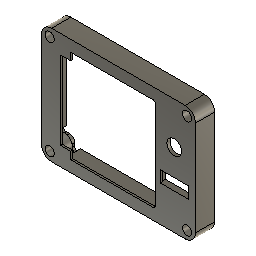
deksel groot projectdoosje v9 (Autodesk Fusion 360 design; units mm, degrees)
Autodesk Fusion 360 part; units mm, degrees
sketch "Sketch1" plane through (0, 0, 0) normal (0, 1, 0) x (1, 0, 0)
  line L0 (8, 0) -> (112, 0)
  line L1 (120, -8) -> (120, -82)
  line L2 (112, -90) -> (8, -90)
  line L3 (0, -82) -> (0, -8)
  arc A0 (0, -82) -> (8, -90) centre (8, -82) ccw
  arc A1 (8, 0) -> (0, -8) centre (8, -8) ccw
  arc A2 (120, -8) -> (112, 0) centre (112, -8) ccw
  arc A3 (112, -90) -> (120, -82) centre (112, -82) ccw
  point P0 (120, 0)
  point P1 (0, -90)
  dimension "d1" = 120
  dimension "d2" = 90
  dimension "d3" = 8
  constraint horizontal L0
  constraint vertical L1
  constraint horizontal L2
  constraint vertical L3
  constraint coincident P1 L2
  constraint coincident P1 L3
  constraint tangent L2 A0
  constraint tangent L3 A0
  constraint coincident origin L0
  constraint coincident origin L3
  constraint tangent L0 A1
  constraint tangent L3 A1
  constraint equal A0 A1
  constraint coincident P0 L0
  constraint coincident P0 L1
  constraint tangent L0 A2
  constraint tangent L1 A2
  constraint equal A0 A2
  constraint tangent L1 A3
  constraint tangent L2 A3
  constraint equal A0 A3
  measures "d1" distance of origin P0
  measures "d2" distance of origin P1
  measures "d3" radius of A0
extrude "Extrude1" add sketch "Sketch1" along normal blind 15
sketch "Sketch2" plane through (0, 0, 0) normal (0, -1, 0) x (1, 0, 0)
  arc A0 (8, 90) -> (0, 82) centre (8, 82) ccw
  line L0 (0, 82) -> (0, 8)
  arc A1 (0, 8) -> (8, 0) centre (8, 8) ccw
  line L1 (8, 0) -> (112, 0)
  arc A2 (112, 0) -> (120, 8) centre (112, 8) ccw
  line L2 (120, 8) -> (120, 82)
  arc A3 (120, 82) -> (112, 90) centre (112, 82) ccw
  line L3 (112, 90) -> (8, 90)
  line L4 (60, 0) -> (60, 90) construction
  line L5 (120, 45) -> (0, 45) construction
  point P0 (6.5, 6.5)
  point P1 (6.5, 83.5)
  point P2 (113.5, 6.5)
  point P3 (113.5, 83.5)
  dimension "d86" = 107
  dimension "d87" = 77
  constraint midpoint L1 L4.start
  constraint midpoint L3 L4.end
  constraint midpoint L2 L5.start
  constraint midpoint L0 L5.end
  constraint symmetric P0 P2 L4
  constraint symmetric P2 P3 L5
  constraint symmetric P0 P1 L5
  measures "d86" distance of P0 P2
  measures "d87" distance of P2 P3
hole "Hole1" at (6.5, 0, 83.5) at (6.5, 0, 6.5) at (113.5, 0, 6.5) at (113.5, 0, 83.5) direction (0, 1, 0) diameter 4 end through all counterbore diameter 7.2 counterbore depth 5
sketch "Sketch3" plane through (0, 0, 0) normal (0, -1, 0) x (1, 0, 0)
  circle A0 centre (113.5, 6.5) radius 3.6
  circle A1 centre (6.5, 83.5) radius 3.6
  circle A2 centre (6.5, 6.5) radius 3.6
  circle A3 centre (113.5, 83.5) radius 3.6
  arc A4 (8, 90) -> (0, 82) centre (8, 82) ccw
  line L0 (0, 82) -> (0, 8)
  arc A5 (0, 8) -> (8, 0) centre (8, 8) ccw
  line L1 (8, 0) -> (112, 0)
  arc A6 (112, 0) -> (120, 8) centre (112, 8) ccw
  line L2 (120, 8) -> (120, 82)
  arc A7 (120, 82) -> (112, 90) centre (112, 82) ccw
  line L3 (112, 90) -> (8, 90)
  circle A8 centre (6.5, 6.5) radius 3
  circle A9 centre (6.5, 83.5) radius 3
  circle A10 centre (113.5, 83.5) radius 3
  circle A11 centre (113.5, 6.5) radius 3
  dimension "d18" = 6
  dimension "d19" = 6
  dimension "d20" = 6
  dimension "d21" = 6
  constraint concentric A2 A8
  constraint concentric A1 A9
  constraint concentric A3 A10
  constraint concentric A0 A11
  measures "d18" diameter of A8
  measures "d19" diameter of A9
  measures "d20" diameter of A10
  measures "d21" diameter of A11
extrude "Extrude2" cut sketch "Sketch3" against normal blind 11 contours A8 | A9 | A10 | A11
sketch "Sketch4" plane through (0, 0, 0) normal (0, -1, 0) x (1, 0, 0)
  circle A0 centre (113.5, 6.5) radius 3.6
  circle A1 centre (6.5, 83.5) radius 3.6
  circle A2 centre (6.5, 6.5) radius 3.6
  circle A3 centre (113.5, 83.5) radius 3.6
  arc A4 (8, 90) -> (0, 82) centre (8, 82) ccw
  line L0 (0, 82) -> (0, 8)
  arc A5 (0, 8) -> (8, 0) centre (8, 8) ccw
  line L1 (8, 0) -> (112, 0)
  arc A6 (112, 0) -> (120, 8) centre (112, 8) ccw
  line L2 (120, 8) -> (120, 82)
  arc A7 (120, 82) -> (112, 90) centre (112, 82) ccw
  line L3 (112, 90) -> (8, 90)
  circle A8 centre (6.5, 6.5) radius 3.5
  line L4 (4.7617, 3.3475) -> (9.6525, 8.2383)
  line L5 (3.3475, 4.7617) -> (8.2383, 9.6525)
  line L6 (60, 90) -> (60, 0) construction
  line L7 (0, 45) -> (120, 45) construction
  circle A9 centre (6.5, 83.5) radius 3.5
  line L8 (4.7617, 86.6525) -> (9.6525, 81.7617)
  line L9 (3.3475, 85.2383) -> (8.2383, 80.3475)
  line L10 (115.2383, 86.6525) -> (110.3475, 81.7617)
  line L11 (116.6525, 85.2383) -> (111.7617, 80.3475)
  circle A10 centre (113.5, 83.5) radius 3.5
  circle A11 centre (113.5, 6.5) radius 3.5
  line L12 (116.6525, 4.7617) -> (111.7617, 9.6525)
  line L13 (115.2383, 3.3475) -> (110.3475, 8.2383)
  dimension "d24" = 45
  dimension "d25" = 2
  dimension "d26" = 1
  dimension "d27" = 6.5
  dimension "d28" = 7
  constraint concentric A2 A8
  constraint coincident A2 L4.start
  constraint coincident A2 L4.end
  constraint coincident A2 L5.start
  constraint coincident A2 L5.end
  constraint parallel L4 L5
  constraint midpoint L3 L6.start
  constraint midpoint L1 L6.end
  constraint midpoint L0 L7.start
  constraint midpoint L2 L7.end
  constraint symmetric A8 L7 A9
  constraint symmetric L4.start L7 L8.start
  constraint symmetric L4.end L7 L8.end
  constraint symmetric L5.start L7 L9.start
  constraint symmetric L5.end L7 L9.end
  constraint symmetric A8 L6 A11
  constraint symmetric L4.start L6 L13.start
  constraint symmetric L4.end L6 L13.end
  constraint symmetric L5.start L6 L12.start
  constraint symmetric L5.end L6 L12.end
  constraint symmetric L6 A9 A10
  constraint symmetric L6 L8.start L10.start
  constraint symmetric L6 L8.end L10.end
  constraint symmetric L6 L9.start L11.start
  constraint symmetric L6 L9.end L11.end
  measures "d24" angle of L1 L4
  measures "d25" distance of L4 L5
  measures "d26" distance of A2.centre L4
  measures "d27" distance of L1 A2.centre
  measures "d28" diameter of A8
extrude "Extrude3" cut sketch "Sketch4" against normal through all contours A11 L12 L13 | A9 L8 L9 | A8 L4 L5 | L10 L11 A10
sketch "Sketch11" plane through (0, 15, 0) normal (0, 1, 0) x (-1, 0, 0)
  line L0 (-116.5788, 4.8354) -> (-115.4319, 5.9824)
  arc A0 (-112.9824, 8.4319) -> (-115.4319, 5.9824) centre (-113.5, 6.5) ccw
  line L1 (-112.9824, 8.4319) -> (-111.8354, 9.5788)
  arc A1 (-110.4212, 8.1646) -> (-111.8354, 9.5788) centre (-113.5, 6.5) ccw
  line L2 (-110.4212, 8.1646) -> (-111.5681, 7.0176)
  arc A2 (-114.0176, 4.5681) -> (-111.5681, 7.0176) centre (-113.5, 6.5) ccw
  line L3 (-114.0176, 4.5681) -> (-115.1646, 3.4212)
  line L4 (-111.8354, 80.4212) -> (-112.9824, 81.5681)
  arc A3 (-115.4319, 84.0176) -> (-112.9824, 81.5681) centre (-113.5, 83.5) ccw
  line L5 (-115.4319, 84.0176) -> (-116.5788, 85.1646)
  arc A4 (-115.1646, 86.5788) -> (-116.5788, 85.1646) centre (-113.5, 83.5) ccw
  line L6 (-115.1646, 86.5788) -> (-114.0176, 85.4319)
  arc A5 (-111.5681, 82.9824) -> (-114.0176, 85.4319) centre (-113.5, 83.5) ccw
  line L7 (-111.5681, 82.9824) -> (-110.4212, 81.8354)
  arc A6 (-111.8354, 80.4212) -> (-110.4212, 81.8354) centre (-113.5, 83.5) ccw
  line L8 (-8.1646, 9.5788) -> (-7.0176, 8.4319)
  arc A7 (-4.5681, 5.9824) -> (-7.0176, 8.4319) centre (-6.5, 6.5) ccw
  line L9 (-4.5681, 5.9824) -> (-3.4212, 4.8354)
  arc A8 (-4.8354, 3.4212) -> (-3.4212, 4.8354) centre (-6.5, 6.5) ccw
  line L10 (-4.8354, 3.4212) -> (-5.9824, 4.5681)
  arc A9 (-8.4319, 7.0176) -> (-5.9824, 4.5681) centre (-6.5, 6.5) ccw
  line L11 (-8.4319, 7.0176) -> (-9.5788, 8.1646)
  arc A10 (-8.1646, 9.5788) -> (-9.5788, 8.1646) centre (-6.5, 6.5) ccw
  line L12 (-3.4212, 85.1646) -> (-4.5681, 84.0176)
  arc A11 (-7.0176, 81.5681) -> (-4.5681, 84.0176) centre (-6.5, 83.5) ccw
  line L13 (-7.0176, 81.5681) -> (-8.1646, 80.4212)
  arc A12 (-9.5788, 81.8354) -> (-8.1646, 80.4212) centre (-6.5, 83.5) ccw
  line L14 (-9.5788, 81.8354) -> (-8.4319, 82.9824)
  arc A13 (-5.9824, 85.4319) -> (-8.4319, 82.9824) centre (-6.5, 83.5) ccw
  line L15 (-5.9824, 85.4319) -> (-4.8354, 86.5788)
  arc A14 (0, 82) -> (-8, 90) centre (-8, 82) ccw
  line L16 (-8, 90) -> (-112, 90)
  arc A15 (-112, 90) -> (-120, 82) centre (-112, 82) ccw
  line L17 (-120, 82) -> (-120, 8)
  arc A16 (-120, 8) -> (-112, 0) centre (-112, 8) ccw
  line L18 (-112, 0) -> (-8, 0)
  arc A17 (-8, 0) -> (0, 8) centre (-8, 8) ccw
  line L19 (0, 8) -> (0, 82)
  line L20 (-120, 45) -> (0, 45) construction
  line L21 (-60, 90) -> (-60, 0) construction
  line L22 (-118.5, 45) -> (-118.5, 79)
  line L23 (-118.5, 79) -> (-113, 79)
  line L24 (-109, 83) -> (-109, 88.5)
  line L25 (-109, 88.5) -> (-60, 88.5)
  arc A18 (-113, 79) -> (-109, 83) centre (-113, 83) ccw
  arc A19 (-116.5788, 4.8354) -> (-115.1646, 3.4212) centre (-113.5, 6.5) ccw
  arc A20 (-3.4212, 85.1646) -> (-4.8354, 86.5788) centre (-6.5, 83.5) ccw
  line L26 (-11, 88.5) -> (-60, 88.5)
  line L27 (-11, 83) -> (-11, 88.5)
  arc A21 (-11, 83) -> (-7, 79) centre (-7, 83) ccw
  line L28 (-1.5, 79) -> (-7, 79)
  line L29 (-1.5, 45) -> (-1.5, 79)
  line L30 (-118.5, 45) -> (-118.5, 11)
  line L31 (-118.5, 11) -> (-113, 11)
  arc A22 (-109, 7) -> (-113, 11) centre (-113, 7) ccw
  line L32 (-109, 7) -> (-109, 1.5)
  line L33 (-109, 1.5) -> (-60, 1.5)
  line L34 (-11, 1.5) -> (-60, 1.5)
  line L35 (-11, 7) -> (-11, 1.5)
  arc A23 (-7, 11) -> (-11, 7) centre (-7, 7) ccw
  line L36 (-1.5, 11) -> (-7, 11)
  line L37 (-1.5, 45) -> (-1.5, 11)
  dimension "d88" = 11
  dimension "d89" = 11
  dimension "d90" = 1.5
  dimension "d91" = 1.5
  dimension "d92" = 4
  constraint midpoint L17 L20.start
  constraint midpoint L19 L20.end
  constraint midpoint L16 L21.start
  constraint midpoint L18 L21.end
  constraint coincident L20 L22.start
  constraint perpendicular L20 L22
  constraint perpendicular L22 L23
  constraint perpendicular L23 L24
  constraint coincident L21 L25.end
  constraint perpendicular L21 L25
  constraint tangent L23 A18
  constraint tangent L24 A18
  constraint symmetric L21 L22.start L29.start
  constraint symmetric L21 L22.end L28.start
  constraint symmetric L21 L24.end L26.start
  constraint symmetric L21 L25.end L26.end
  constraint symmetric L21 L23.end A21.end
  constraint symmetric L21 L24.start L27.start
  constraint symmetric L21 A18 A21
  constraint symmetric L20 L22.start L30.start
  constraint symmetric L20 L22.end L30.end
  constraint symmetric L20 L24.end L32.end
  constraint symmetric L20 L25.end L33.end
  constraint symmetric L20 L23.end L31.end
  constraint symmetric L20 L24.start A22.start
  constraint symmetric L20 A18 A22
  constraint symmetric L20 L26.start L34.start
  constraint symmetric L20 L27.start L35.start
  constraint symmetric L20 A21.end A23.start
  constraint symmetric L20 A21 A23
  constraint symmetric L20 L28.start L36.start
  constraint symmetric L20 L29.start L37.start
  measures "d88" distance of L17 L24
  measures "d89" distance of L16 L23
  measures "d90" distance of L16 L25
  measures "d91" distance of L17 L22
  measures "d92" radius of A18
extrude "Extrude9" cut sketch "Sketch11" against normal up to surface (13.5 mm away) contours L22 L23 L24 L25 A18 L26 L27 A21 L28 L29 L30 L31 A22 L32 L33 L34 L35 A23 L36 L37
sketch "Sketch15" plane through (0, 1.5, 0) normal (0, 1, 0) x (-1, 0, 0)
  arc A0 (-11, 83) -> (-7, 79) centre (-7, 83) ccw
  line L0 (-11, 83) -> (-11, 88.5)
  line L1 (-11, 88.5) -> (-109, 88.5)
  line L2 (-109, 88.5) -> (-109, 83)
  arc A1 (-113, 79) -> (-109, 83) centre (-113, 83) ccw
  line L3 (-113, 79) -> (-118.5, 79)
  line L4 (-118.5, 79) -> (-118.5, 11)
  line L5 (-118.5, 11) -> (-113, 11)
  arc A2 (-109, 7) -> (-113, 11) centre (-113, 7) ccw
  line L6 (-109, 7) -> (-109, 1.5)
  line L7 (-109, 1.5) -> (-11, 1.5)
  line L8 (-11, 1.5) -> (-11, 7)
  arc A3 (-7, 11) -> (-11, 7) centre (-7, 7) ccw
  line L9 (-7, 11) -> (-1.5, 11)
  line L10 (-1.5, 11) -> (-1.5, 79)
  line L11 (-1.5, 79) -> (-7, 79)
  line L12 (-11, 1.5) -> (-109, 1.5)
  line L13 (-109, 1.5) -> (-109, 3.5)
  line L14 (-105, 3.5) -> (-14.9861, 3.5)
  line L15 (-11, 3.5) -> (-11, 1.5)
  line L16 (-118.5, 11) -> (-116.5, 11)
  line L17 (-116.5, 15) -> (-116.5, 75)
  line L18 (-116.5, 79) -> (-118.5, 79)
  line L19 (-118.5, 79) -> (-118.5, 11)
  line L20 (-11, 88.5) -> (-109, 88.5)
  line L21 (-109, 88.5) -> (-109, 86.5)
  line L22 (-105, 86.5) -> (-15, 86.5)
  line L23 (-11, 86.5) -> (-11, 88.5)
  line L24 (-1.5, 11) -> (-3.5, 11)
  line L25 (-3.5, 15) -> (-3.5, 75)
  line L26 (-3.5, 79) -> (-1.5, 79)
  line L27 (-1.5, 79) -> (-1.5, 11)
  line L28 (-5.5, 13) -> (-6, 13)
  line L29 (-13, 6) -> (-13, 3.5)
  arc A4 (-6, 13) -> (-12.9892, 5.6111) centre (-6, 6) ccw
  line L30 (-60, 3.5) -> (-60, 86.5) construction
  line L31 (-107, 6) -> (-107, 5.5)
  arc A5 (-107, 6) -> (-114, 13) centre (-114, 6) ccw
  line L32 (-114.5, 13) -> (-114, 13)
  line L33 (-3.5, 45) -> (-116.5, 45)
  line L34 (-13, 84) -> (-13, 84.5)
  arc A6 (-13, 84) -> (-6, 77) centre (-6, 84) ccw
  line L35 (-5.5, 77) -> (-6, 77)
  line L36 (-107, 84) -> (-107, 84.5)
  arc A7 (-114, 77) -> (-107, 84) centre (-114, 84) ccw
  line L37 (-114.5, 77) -> (-114, 77)
  arc A8 (-14.9861, 3.5) -> (-12.9892, 5.6111) centre (-14.9861, 5.5) ccw
  arc A9 (-5.5, 13) -> (-3.5, 15) centre (-5.5, 15) ccw
  arc A10 (-3.5, 75) -> (-5.5, 77) centre (-5.5, 75) ccw
  arc A11 (-13, 84.5) -> (-15, 86.5) centre (-15, 84.5) ccw
  arc A12 (-105, 86.5) -> (-107, 84.5) centre (-105, 84.5) ccw
  arc A13 (-114.5, 77) -> (-116.5, 75) centre (-114.5, 75) ccw
  arc A14 (-116.5, 15) -> (-114.5, 13) centre (-114.5, 15) ccw
  arc A15 (-107, 5.5) -> (-105, 3.5) centre (-105, 5.5) ccw
  dimension "d109" = 2
  dimension "d110" = 2
  dimension "d111" = 2
  dimension "d112" = 2
  dimension "d115" = 2
  dimension "d116" = 2
  dimension "d117" = 7
  dimension "d118" = 2
  constraint horizontal L12
  constraint vertical L13
  constraint horizontal L14
  constraint vertical L15
  constraint coincident L6 L13.end
  constraint coincident L7.end L8.start
  constraint horizontal L16
  constraint vertical L17
  constraint horizontal L18
  constraint vertical L19
  constraint coincident L3 L18.start
  constraint coincident L4.end L5.start
  constraint horizontal L20
  constraint vertical L21
  constraint horizontal L22
  constraint vertical L23
  constraint coincident L2 L21.end
  constraint coincident L0.end L1.start
  constraint horizontal L24
  constraint vertical L25
  constraint horizontal L26
  constraint vertical L27
  constraint coincident L11 L26.start
  constraint coincident L9.end L10.start
  constraint perpendicular L25 L28
  constraint coincident L14 L29.end
  constraint perpendicular L14 L29
  constraint tangent L28 A4
  constraint tangent L29 A4
  constraint symmetric L28.end L30 A5.end
  constraint symmetric L29.start L30 L31.start
  constraint symmetric A4 L30 A5
  constraint symmetric L28.end L33 A6.end
  constraint symmetric L29.start L33 L34.start
  constraint symmetric A4 L33 A6
  constraint symmetric L31.start L33 L36.start
  constraint symmetric A5.end L33 A7.start
  constraint symmetric A5 L33 A7
  constraint coincident L14 L30.start
  constraint tangent L14 A8
  constraint tangent A4 A8
  constraint coincident L25 L33.start
  constraint coincident L24.end L25
  constraint tangent L28 A9
  constraint tangent L25 A9
  constraint equal A8 A9
  constraint coincident L26.start L25
  constraint tangent L35 A10
  constraint tangent L25 A10
  constraint equal A8 A10
  constraint coincident L22 L30.end
  constraint coincident L23.start L22
  constraint tangent L34 A11
  constraint tangent L22 A11
  constraint equal A8 A11
  constraint coincident L21.end L22
  constraint tangent L36 A12
  constraint tangent L22 A12
  constraint equal A8 A12
  constraint coincident L17 L33.end
  constraint coincident L18.start L17
  constraint tangent L37 A13
  constraint tangent L17 A13
  constraint equal A8 A13
  constraint coincident L16.end L17
  constraint tangent L17 A14
  constraint tangent L32 A14
  constraint equal A8 A14
  constraint coincident L13.end L14
  constraint tangent L14 A15
  constraint tangent L31 A15
  constraint equal A8 A15
  measures "d109" distance of L12 L14
  measures "d110" distance of L17 L19
  measures "d111" distance of L20 L22
  measures "d112" distance of L25 L27
  measures "d115" distance of L8 L29
  measures "d116" distance of L9 L28
  measures "d117" radius of A4
  measures "d118" radius of A8
extrude "Extrude13" add sketch "Sketch15" along normal up to surface (10 mm away)
fillet "Fillet2" radius 3 8 edges at (11, 13.25, 1.5) (1.5, 13.25, 11) (109, 13.25, 1.5) (118.5, 13.25, 11) (109, 13.25, 88.5) (118.5, 13.25, 79) (11, 13.25, 88.5) (1.5, 13.25, 79)
sketch "Sketch16" plane through (0, 1.5, 0) normal (0, 1, 0) x (-1, 0, 0)
  arc A0 (-107, 6) -> (-114, 13) centre (-114, 6) ccw
  line L0 (-107, 6) -> (-107, 5.5)
  arc A1 (-107, 5.5) -> (-105, 3.5) centre (-105, 5.5) ccw
  line L1 (-105, 3.5) -> (-14.9861, 3.5)
  arc A2 (-14.9861, 3.5) -> (-12.9892, 5.6111) centre (-14.9861, 5.5) ccw
  arc A3 (-6, 13) -> (-12.9892, 5.6111) centre (-6, 6) ccw
  line L2 (-6, 13) -> (-5.5, 13)
  arc A4 (-5.5, 13) -> (-3.5, 15) centre (-5.5, 15) ccw
  line L3 (-3.5, 15) -> (-3.5, 75)
  arc A5 (-3.5, 75) -> (-5.5, 77) centre (-5.5, 75) ccw
  line L4 (-5.5, 77) -> (-6, 77)
  arc A6 (-13, 84) -> (-6, 77) centre (-6, 84) ccw
  line L5 (-13, 84) -> (-13, 84.5)
  arc A7 (-13, 84.5) -> (-15, 86.5) centre (-15, 84.5) ccw
  line L6 (-15, 86.5) -> (-105, 86.5)
  arc A8 (-105, 86.5) -> (-107, 84.5) centre (-105, 84.5) ccw
  line L7 (-107, 84.5) -> (-107, 84)
  arc A9 (-114, 77) -> (-107, 84) centre (-114, 84) ccw
  line L8 (-114, 77) -> (-114.5, 77)
  arc A10 (-114.5, 77) -> (-116.5, 75) centre (-114.5, 75) ccw
  line L9 (-116.5, 75) -> (-116.5, 15)
  arc A11 (-116.5, 15) -> (-114.5, 13) centre (-114.5, 15) ccw
  line L10 (-114.5, 13) -> (-114, 13)
  line L11 (-104.5, 86.5) -> (-15.5, 86.5)
  line L12 (-15.5, 86.5) -> (-15.5, 85)
  line L13 (-15.5, 85) -> (-104.5, 85)
  line L14 (-104.5, 85) -> (-104.5, 86.5)
  line L15 (-3.5, 74.5) -> (-5, 74.5)
  line L16 (-5, 74.5) -> (-5, 15.5)
  line L17 (-5, 15.5) -> (-3.5, 15.5)
  line L18 (-3.5, 15.5) -> (-3.5, 74.5)
  line L19 (-15.5, 3.5) -> (-104.5, 3.5)
  line L20 (-104.5, 3.5) -> (-104.5, 5)
  line L21 (-104.5, 5) -> (-15.5, 5)
  line L22 (-15.5, 5) -> (-15.5, 3.5)
  line L23 (-116.5, 74.5) -> (-115, 74.5)
  line L24 (-115, 74.5) -> (-115, 15.5)
  line L25 (-115, 15.5) -> (-116.5, 15.5)
  line L26 (-116.5, 15.5) -> (-116.5, 74.5)
  line L27 (-103.8997, 85) -> (-104.5, 85)
  line L28 (-115, 74.5) -> (-115, 74)
  line L29 (-115, 45) -> (-5, 45) construction
  line L30 (-60, 85) -> (-60, 5) construction
  dimension "d121" = 1.5
  dimension "d122" = 12
  dimension "d123" = 12
  dimension "d124" = 1.5
  dimension "d125" = 12
  dimension "d126" = 12
  dimension "d127" = 12
  dimension "d128" = 1.5
  dimension "d129" = 12
  dimension "d130" = 1.5
  dimension "d131" = 12
  dimension "d132" = 12
  constraint horizontal L11
  constraint vertical L12
  constraint horizontal L13
  constraint vertical L14
  constraint coincident L6 L11.start
  constraint horizontal L15
  constraint vertical L16
  constraint horizontal L17
  constraint vertical L18
  constraint coincident L3 L15.start
  constraint horizontal L19
  constraint vertical L20
  constraint horizontal L21
  constraint vertical L22
  constraint coincident L1 L19.start
  constraint horizontal L23
  constraint vertical L24
  constraint horizontal L25
  constraint vertical L26
  constraint coincident L9 L23.start
  constraint horizontal L27
  constraint perpendicular L23 L28
  constraint midpoint L24 L29.start
  constraint midpoint L16 L29.end
  constraint midpoint L13 L30.start
  constraint midpoint L21 L30.end
  measures "d121" distance of L11 L13
  measures "d122" distance of L9 L14
  measures "d123" distance of L3 L12
  measures "d124" distance of L16 L18
  measures "d125" distance of L11 L15
  measures "d126" distance of L1 L17
  measures "d127" distance of L18 L22
  measures "d128" distance of L19 L21
  measures "d129" distance of L9 L19.end
  measures "d130" distance of L24 L26
  measures "d131" distance of L19 L24.end
  measures "d132" distance of L11 L23.end
extrude "Extrude14" add sketch "Sketch16" along normal up to surface (13.5 mm away) contours L1 L19 L20 L21 L22 | L9 L23 L24 L25 L26 L28 | L3 L15 L16 L17 L18 | L6 L11 L12 L13 L14 L27
sketch "Sketch17" plane through (0, 0, 0) normal (0, -1, 0) x (1, 0, 0)
  circle A0 centre (113.5, 6.5) radius 3.6
  circle A1 centre (6.5, 83.5) radius 3.6
  circle A2 centre (6.5, 6.5) radius 3.6
  circle A3 centre (113.5, 83.5) radius 3.6
  arc A4 (8, 90) -> (0, 82) centre (8, 82) ccw
  line L0 (0, 82) -> (0, 8)
  arc A5 (0, 8) -> (8, 0) centre (8, 8) ccw
  line L1 (8, 0) -> (112, 0)
  arc A6 (112, 0) -> (120, 8) centre (112, 8) ccw
  line L2 (120, 8) -> (120, 82)
  arc A7 (120, 82) -> (112, 90) centre (112, 82) ccw
  line L3 (112, 90) -> (8, 90)
  line L4 (15, 81.25) -> (87, 81.25)
  line L5 (89, 79.25) -> (89, 10.75)
  line L6 (87, 8.75) -> (15, 8.75)
  line L7 (15, 8.75) -> (15, 81.25)
  line L8 (15, 81.25) -> (23, 81.25)
  line L9 (23, 81.25) -> (23, 75.5)
  line L10 (23, 75.5) -> (15, 75.5)
  line L11 (15, 75.5) -> (15, 81.25)
  line L12 (15, 8.75) -> (23, 8.75)
  line L13 (23, 8.75) -> (23, 14.5)
  line L14 (23, 14.5) -> (15, 14.5)
  line L15 (15, 14.5) -> (15, 8.75)
  arc A8 (87, 8.75) -> (89, 10.75) centre (87, 10.75) ccw
  arc A9 (89, 79.25) -> (87, 81.25) centre (87, 79.25) ccw
  line L16 (0, 45) -> (120, 45) construction
  point P0 (89, 8.75)
  dimension "d140" = 72.5
  dimension "d141" = 74
  dimension "d143" = 8
  dimension "d145" = 2
  dimension "d146" = 15
  dimension "d166" = 61
  dimension "d167" = 66
  constraint horizontal L4
  constraint vertical L5
  constraint horizontal L6
  constraint vertical L7
  constraint horizontal L8
  constraint vertical L9
  constraint horizontal L10
  constraint vertical L11
  constraint horizontal L12
  constraint vertical L13
  constraint horizontal L14
  constraint vertical L15
  constraint collinear L9 L13
  constraint coincident P0 L5
  constraint coincident P0 L6
  constraint tangent L5 A8
  constraint tangent L6 A8
  constraint tangent L4 A9
  constraint tangent L5 A9
  constraint equal A8 A9
  constraint midpoint L0 L16.start
  constraint midpoint L2 L16.end
  constraint symmetric L4 L6 L16
  constraint equal L9 L13
  measures "d140" distance of L4 L6
  measures "d141" distance of P0 L6.end
  measures "d143" distance of L9.end L10.end
  measures "d145" radius of A8
  measures "d146" distance of L0 L7
  measures "d166" distance of L10 L14
  measures "d167" distance of L5 L9
extrude "Extrude15" cut sketch "Sketch17" against normal through all contours L4 L5 L6 L7 L9 L10 L13 L14 A8 A9
sketch "Sketch22" plane through (0, 1.5, 0) normal (0, 1, 0) x (-1, 0, 0)
  line L0 (-15, 75.5) -> (-15, 14.5)
  line L1 (-15, 14.5) -> (-23, 14.5)
  line L2 (-23, 14.5) -> (-23, 8.75)
  line L3 (-23, 8.75) -> (-87, 8.75)
  arc A0 (-89, 10.75) -> (-87, 8.75) centre (-87, 10.75) ccw
  line L4 (-89, 10.75) -> (-89, 79.25)
  arc A1 (-87, 81.25) -> (-89, 79.25) centre (-87, 79.25) ccw
  line L5 (-87, 81.25) -> (-23, 81.25)
  line L6 (-23, 81.25) -> (-23, 75.5)
  line L7 (-23, 75.5) -> (-15, 75.5)
  line L8 (-15.5, 5) -> (-15.5, 3.5)
  line L9 (-15.5, 3.5) -> (-14.9861, 3.5)
  arc A2 (-14.9861, 3.5) -> (-12.9892, 5.6111) centre (-14.9861, 5.5) ccw
  arc A3 (-6, 13) -> (-12.9892, 5.6111) centre (-6, 6) ccw
  line L10 (-6, 13) -> (-5.5, 13)
  arc A4 (-5.5, 13) -> (-3.5, 15) centre (-5.5, 15) ccw
  line L11 (-3.5, 15) -> (-3.5, 15.5)
  line L12 (-3.5, 15.5) -> (-5, 15.5)
  line L13 (-5, 15.5) -> (-5, 74.5)
  line L14 (-5, 74.5) -> (-3.5, 74.5)
  line L15 (-3.5, 74.5) -> (-3.5, 75)
  arc A5 (-3.5, 75) -> (-5.5, 77) centre (-5.5, 75) ccw
  line L16 (-5.5, 77) -> (-6, 77)
  arc A6 (-13, 84) -> (-6, 77) centre (-6, 84) ccw
  line L17 (-13, 84) -> (-13, 84.5)
  arc A7 (-13, 84.5) -> (-15, 86.5) centre (-15, 84.5) ccw
  line L18 (-15, 86.5) -> (-15.5, 86.5)
  line L19 (-15.5, 86.5) -> (-15.5, 85)
  line L20 (-15.5, 85) -> (-104.5, 85)
  line L21 (-104.5, 85) -> (-104.5, 86.5)
  line L22 (-104.5, 86.5) -> (-105, 86.5)
  arc A8 (-105, 86.5) -> (-107, 84.5) centre (-105, 84.5) ccw
  line L23 (-107, 84.5) -> (-107, 84)
  arc A9 (-114, 77) -> (-107, 84) centre (-114, 84) ccw
  line L24 (-114, 77) -> (-114.5, 77)
  arc A10 (-114.5, 77) -> (-116.5, 75) centre (-114.5, 75) ccw
  line L25 (-116.5, 75) -> (-116.5, 74.5)
  line L26 (-116.5, 74.5) -> (-115, 74.5)
  line L27 (-115, 74.5) -> (-115, 15.5)
  line L28 (-115, 15.5) -> (-116.5, 15.5)
  line L29 (-116.5, 15.5) -> (-116.5, 15)
  arc A11 (-116.5, 15) -> (-114.5, 13) centre (-114.5, 15) ccw
  line L30 (-114.5, 13) -> (-114, 13)
  arc A12 (-107, 6) -> (-114, 13) centre (-114, 6) ccw
  line L31 (-107, 6) -> (-107, 5.5)
  arc A13 (-107, 5.5) -> (-105, 3.5) centre (-105, 5.5) ccw
  line L32 (-105, 3.5) -> (-104.5, 3.5)
  line L33 (-104.5, 3.5) -> (-104.5, 5)
  line L34 (-104.5, 5) -> (-15.5, 5)
  line L35 (-89, 5) -> (-92, 5)
  line L36 (-92, 5) -> (-92, 85)
  line L37 (-92, 85) -> (-89, 85)
  line L38 (-89, 85) -> (-89, 5)
  dimension "d162" = 3
  constraint horizontal L35
  constraint vertical L36
  constraint horizontal L37
  constraint vertical L38
  constraint coincident L20 L36.end
  constraint coincident L34 L35.start
  constraint collinear L4 L38
  measures "d162" distance of L36 L38
extrude "Extrude19" add sketch "Sketch22" along normal blind 3 contours L4 L20 L34 L35 L36 L37 L38
sketch "Sketch23" plane through (0, 0, 0) normal (0, -1, 0) x (1, 0, 0)
  line L0 (15, 14.5) -> (15, 75.5)
  line L1 (15, 75.5) -> (23, 75.5)
  line L2 (23, 75.5) -> (23, 81.25)
  line L3 (23, 81.25) -> (87, 81.25)
  arc A0 (89, 79.25) -> (87, 81.25) centre (87, 79.25) ccw
  line L4 (89, 79.25) -> (89, 10.75)
  arc A1 (87, 8.75) -> (89, 10.75) centre (87, 10.75) ccw
  line L5 (87, 8.75) -> (23, 8.75)
  line L6 (23, 8.75) -> (23, 14.5)
  line L7 (23, 14.5) -> (15, 14.5)
  circle A2 centre (113.5, 6.5) radius 3.6
  circle A3 centre (6.5, 83.5) radius 3.6
  circle A4 centre (6.5, 6.5) radius 3.6
  circle A5 centre (113.5, 83.5) radius 3.6
  arc A6 (8, 90) -> (0, 82) centre (8, 82) ccw
  line L8 (0, 82) -> (0, 8)
  arc A7 (0, 8) -> (8, 0) centre (8, 8) ccw
  line L9 (8, 0) -> (112, 0)
  arc A8 (112, 0) -> (120, 8) centre (112, 8) ccw
  line L10 (120, 8) -> (120, 82)
  arc A9 (120, 82) -> (112, 90) centre (112, 82) ccw
  line L11 (112, 90) -> (8, 90)
  line L12 (92.5, 37) -> (114.5, 37)
  line L13 (114.5, 37) -> (114.5, 28)
  line L14 (114.5, 28) -> (92.5, 28)
  line L15 (92.5, 28) -> (92.5, 37)
  circle A10 centre (103.5, 57.5) radius 5.75
  line L16 (92.5, 32.5) -> (114.5, 32.5) construction
  line L17 (120, 45) -> (89, 45) construction
  line L18 (115, 74.5) -> (115, 15.5)
  line L19 (92, 85) -> (92, 5)
  line L20 (92, 85) -> (92, 5)
  line L21 (92, 5) -> (92, 85)
  line L22 (92, 5) -> (92, 85)
  line L23 (92, 85) -> (104.5, 85)
  dimension "d172" = 11.5
  dimension "d192" = 23
  dimension "d193" = 22
  dimension "d194" = 0.5
  dimension "d195" = 9
  dimension "d196" = 25
  dimension "d197" = 80
  dimension "d198" = 27.5
  dimension "d199" = 11.5
  constraint horizontal L12
  constraint vertical L13
  constraint horizontal L14
  constraint vertical L15
  constraint midpoint L15 L16.start
  constraint midpoint L13 L16.end
  constraint midpoint L10 L17.start
  constraint midpoint L4 L17.end
  measures "d172" diameter of A10
  measures "d192" distance of L18 L21
  measures "d193" distance of L12.start L12.end
  measures "d194" distance of L13 L18
  measures "d195" distance of L12.end L13.end
  measures "d196" distance of A10.centre L16
  measures "d197" distance of L19.end L19.start
  measures "d198" distance of A10.centre L23
  measures "d199" distance of A10.centre L19
extrude "Extrude20" cut sketch "Sketch23" against normal through all contours L12 L13 L14 L15 | A10
sketch "Sketch24" plane through (0, 1.5, 0) normal (0, 1, 0) x (-1, 0, 0)
  line L0 (-92, 37) -> (-115, 37)
  line L1 (-115, 37) -> (-115, 39)
  line L2 (-115, 39) -> (-92, 39)
  line L3 (-92, 39) -> (-92, 37)
  line L4 (-114.5, 37) -> (-92.5, 37)
  line L5 (-92, 28) -> (-115, 28)
  line L6 (-115, 28) -> (-115, 26)
  line L7 (-115, 26) -> (-92, 26)
  line L8 (-92, 26) -> (-92, 28)
  line L9 (-92.5, 28) -> (-114.5, 28)
  line L10 (-115, 74.5) -> (-115, 15.5)
  line L11 (-92, 85) -> (-92, 5)
  line L12 (-92.5, 37) -> (-92.5, 28)
  dimension "d183" = 2
  dimension "d184" = 2
  dimension "d185" = 0.5
  constraint horizontal L0
  constraint vertical L1
  constraint horizontal L2
  constraint vertical L3
  constraint collinear L0 L4
  constraint horizontal L5
  constraint vertical L6
  constraint horizontal L7
  constraint vertical L8
  constraint collinear L5 L9
  constraint collinear L6 L10
  constraint collinear L8 L11
  measures "d183" distance of L0 L2
  measures "d184" distance of L5 L7
  measures "d185" distance of L11 L12
extrude "Extrude21" add sketch "Sketch24" along normal blind 3 contours L0 L1 L2 L3 L4 L10 L11 | L5 L6 L7 L8 L9 L10 L11
sketch "Sketch25" plane through (0, 1.5, 0) normal (0, 1, 0) x (-1, 0, 0)
  line L0 (-92, 85) -> (-104.5, 85)
  line L1 (-104.5, 86.5) -> (-105, 86.5)
  circle A0 centre (-103.5, 57.5) radius 5.75
  circle A1 centre (-103.5, 57.5) radius 9
  line L2 (-115, 39) -> (-92, 39)
  line L3 (-92, 39) -> (-92, 85)
  line L4 (-104.5, 85) -> (-104.5, 86.5)
  arc A2 (-105, 86.5) -> (-107, 84.5) centre (-105, 84.5) ccw
  line L5 (-107, 84.5) -> (-107, 84)
  arc A3 (-114, 77) -> (-107, 84) centre (-114, 84) ccw
  line L6 (-114, 77) -> (-114.5, 77)
  arc A4 (-114.5, 77) -> (-116.5, 75) centre (-114.5, 75) ccw
  line L7 (-116.5, 75) -> (-116.5, 74.5)
  line L8 (-116.5, 74.5) -> (-115, 74.5)
  line L9 (-115, 74.5) -> (-115, 39)
  circle A5 centre (-103.5, 57.5) radius 5.75
  dimension "d180" = 18
  constraint coincident A0.centre A1.centre
  measures "d180" diameter of A1
extrude "Extrude22" add sketch "Sketch25" along normal blind 1 contours A1
equation "d7 = 7 mm"
equation "d8 = d7"
equation "d9 = d8"
equation "d10 = d9"
equation "d67 = 10.5 mm"
equation "d68 = d67"
equation "d69 = d68"
equation "d89 = d88"
equation "d91 = d90"
equation "d110 = d109"
equation "d111 = d109"
equation "d112 = d109"
equation "d115 = d109"
equation "d116 = d115"
equation "d123 = d122"
equation "d124 = d121"
equation "d125 = d123"
equation "d126 = d125"
equation "d127 = d126"
equation "d128 = d124"
equation "d129 = d123"
equation "d130 = d121"
equation "d131 = d129"
equation "d132 = d122"
equation "d184 = d183"
equation "d194 = ( d192 - d193 ) / 2"
equation "d198 = ( d197 - d196 ) / 2"
equation "d199 = d192 / 2"
